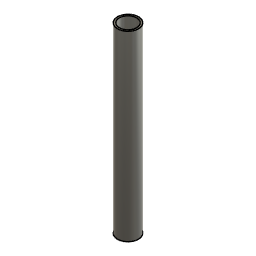
shellnothreads v2 (Autodesk Fusion 360 design; units mm, degrees)
Autodesk Fusion 360 part; units mm, degrees
cylinder "CylinderPrimitive1" add diameter 11.5 height 100 placed x (1, 0, 0) y (0, 0, -1) z (0, 1, 0) at (0, 0, 0)
shell "Shell1" thickness 1 removed faces 1 at (-0.9583, 100, -0.9474)
